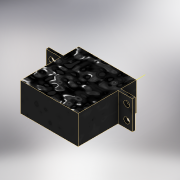
# Autodesk Inventor part: Servo
Saved by Autodesk Inventor 2021 (Build 250183000, 183)
## iProperties
Created: 2024-03-17
Part Number: Servo
Material: PLA
Document SubType Name: Modeling
Designer: Martin
Density: 1.27 g/cm^3
Appearance: PLA
Mass: 42.079 g
Surface Area: 72.9716 cm^2
Volume: 33.1331 cm^3
Author: Martin
Autodesk Inventor part; units mm, degrees
ref_plane "YZ Plane" through (0, 0, 0) normal (1, 0, 0) x (0, 1, 0)
ref_plane "XZ Plane" through (0, 0, 0) normal (0, 1, 0) x (-1, 0, 0)
ref_plane "XY Plane" through (0, 0, 0) normal (0, 0, 1) x (1, 0, 0)
sketch "Sketch1" plane through (0, 0, 0) normal (0, 1, 0) x (-1, 0, 0)
  line L0 (-20, 0) -> (20, 0)
  line L1 (20, 0) -> (20, -40.5)
  line L2 (20, -40.5) -> (-20, -40.5)
  line L3 (-20, -40.5) -> (-20, 0)
  point P0 (0, 0)
  point P1 (0, -40.5)
  dimension "d0" = 40
  dimension "d1" = 40.5
  constraints: 8 end point, 2 parallel, 1 horizontal, 1 midpoint, 1 perpendicular
  measures "d0" distance of L1.end L2.end
  measures "d1" distance of L0.end L1.end
extrude "Extrusion1" add sketch "Sketch1" along normal blind 20
sketch "Sketch2" plane through (20, 0, 0) normal (1, 0, 0) x (0, 0, -1)
  line L0 (27.7, 20) -> (29.7, 20)
  line L1 (29.7, 20) -> (29.7, 0)
  line L2 (29.7, 0) -> (27.7, 0)
  line L3 (27.7, 0) -> (27.7, 20)
  line L4 (40.5, 0) -> (40.5, 20) projected
  line L5 (0, 0) -> (0, 20) projected
  dimension "d4" = 2
  dimension "d31" = 27.7
  constraints: 8 end point, 2 parallel, 1 horizontal, 1 perpendicular
  measures "d4" distance of L1.end L2.end
  measures "d31" distance between parallel lines of L3 L5
extrude "Extrusion2" add sketch "Sketch2" along normal blind 10
sketch "Sketch3" plane through (20, 0, -29.7) normal (0, 0, -1) x (-1, 0, 0)
  circle A0 centre (-6, 15) radius 2
  line L0 (-10, 20) -> (-10, 0) projected
  line L1 (-10, 10) -> (0, 10)
  circle A1 centre (-6, 5) radius 2
  point P0 (20, 0)
  point P1 (-10, 5)
  point P2 (-8, 3.2679)
  dimension "d9" = 4
  dimension "d13" = 5
  dimension "d32" = 4
  constraints: 2 centre point, 2 end point, 1 horizontal, 1 midpoint, 1 symmetric about line, 1 other
  measures "d9" diameter of A0
  measures "d13" distance from line of A0.centre L1
  measures "d32" distance from line of L0 A0.centre
extrude "Extrusion3" cut sketch "Sketch3" against normal up to next
sketch "Sketch4" plane through (20, 0, -40.5) normal (0, 0, -1) x (-1, 0, 0)
  circle A0 centre (10, 10) radius 3
  line L0 (0, 0) -> (0, 20) projected
  line L1 (0, 20) -> (40, 20) projected
  point P0 (20, 0)
  dimension "d16" = 6
  dimension "d17" = 10
  dimension "d18" = 10
  constraints: 1 centre point
  measures "d16" diameter of A0
  measures "d17" distance from line of L0 A0.centre
  measures "d18" distance from line of L1 A0.centre
extrude "Extrusion4" add sketch "Sketch4" along normal blind 6
sketch "Sketch5" plane through (10, 10, -46.5) normal (0, 0, -1) x (-1, 0, 0)
  circle A0 centre (0, 0) radius 3 projected
  line L0 (2.75, -0.1872) -> (3.25, -0.1872)
  line L1 (3.25, -0.1872) -> (3.25, 0.1872)
  line L2 (3.25, 0.1872) -> (2.75, 0.1872)
  line L3 (2.75, 0.1872) -> (2.75, -0.1872)
  line L4 (2.75, -0.1872) -> (3.25, 0.1872) construction
  line L5 (3.25, -0.1872) -> (2.75, 0.1872) construction
  line L6 (2.5575, 1.0279) -> (2.6733, 0.6717)
  line L7 (3.0331, 1.1824) -> (2.5575, 1.0279)
  line L8 (3.1488, 0.8262) -> (3.0331, 1.1824)
  line L9 (2.6733, 0.6717) -> (3.1488, 0.8262)
  line L10 (2.1147, 1.7679) -> (2.3348, 1.4649)
  line L11 (2.5193, 2.0618) -> (2.1147, 1.7679)
  line L12 (2.7394, 1.7588) -> (2.5193, 2.0618)
  line L13 (2.3348, 1.4649) -> (2.7394, 1.7588)
  line L14 (1.4649, 2.3348) -> (1.7679, 2.1147)
  line L15 (1.7588, 2.7394) -> (1.4649, 2.3348)
  line L16 (2.0618, 2.5193) -> (1.7588, 2.7394)
  line L17 (1.7679, 2.1147) -> (2.0618, 2.5193)
  line L18 (0.6717, 2.6733) -> (1.0279, 2.5575)
  line L19 (0.8262, 3.1488) -> (0.6717, 2.6733)
  line L20 (1.1824, 3.0331) -> (0.8262, 3.1488)
  line L21 (1.0279, 2.5575) -> (1.1824, 3.0331)
  line L22 (-0.1872, 2.75) -> (0.1872, 2.75)
  line L23 (-0.1872, 3.25) -> (-0.1872, 2.75)
  line L24 (0.1872, 3.25) -> (-0.1872, 3.25)
  line L25 (0.1872, 2.75) -> (0.1872, 3.25)
  line L26 (-1.0279, 2.5575) -> (-0.6717, 2.6733)
  line L27 (-1.1824, 3.0331) -> (-1.0279, 2.5575)
  line L28 (-0.8262, 3.1488) -> (-1.1824, 3.0331)
  line L29 (-0.6717, 2.6733) -> (-0.8262, 3.1488)
  line L30 (-1.7679, 2.1147) -> (-1.4649, 2.3348)
  line L31 (-2.0618, 2.5193) -> (-1.7679, 2.1147)
  line L32 (-1.7588, 2.7394) -> (-2.0618, 2.5193)
  line L33 (-1.4649, 2.3348) -> (-1.7588, 2.7394)
  line L34 (-2.3348, 1.4649) -> (-2.1147, 1.7679)
  line L35 (-2.7394, 1.7588) -> (-2.3348, 1.4649)
  line L36 (-2.5193, 2.0618) -> (-2.7394, 1.7588)
  line L37 (-2.1147, 1.7679) -> (-2.5193, 2.0618)
  line L38 (-2.6733, 0.6717) -> (-2.5575, 1.0279)
  line L39 (-3.1488, 0.8262) -> (-2.6733, 0.6717)
  line L40 (-3.0331, 1.1824) -> (-3.1488, 0.8262)
  line L41 (-2.5575, 1.0279) -> (-3.0331, 1.1824)
  line L42 (-2.75, -0.1872) -> (-2.75, 0.1872)
  line L43 (-3.25, -0.1872) -> (-2.75, -0.1872)
  line L44 (-3.25, 0.1872) -> (-3.25, -0.1872)
  line L45 (-2.75, 0.1872) -> (-3.25, 0.1872)
  line L46 (-2.5575, -1.0279) -> (-2.6733, -0.6717)
  line L47 (-3.0331, -1.1824) -> (-2.5575, -1.0279)
  line L48 (-3.1488, -0.8262) -> (-3.0331, -1.1824)
  line L49 (-2.6733, -0.6717) -> (-3.1488, -0.8262)
  line L50 (-2.1147, -1.7679) -> (-2.3348, -1.4649)
  line L51 (-2.5193, -2.0618) -> (-2.1147, -1.7679)
  line L52 (-2.7394, -1.7588) -> (-2.5193, -2.0618)
  line L53 (-2.3348, -1.4649) -> (-2.7394, -1.7588)
  line L54 (-1.4649, -2.3348) -> (-1.7679, -2.1147)
  line L55 (-1.7588, -2.7394) -> (-1.4649, -2.3348)
  line L56 (-2.0618, -2.5193) -> (-1.7588, -2.7394)
  line L57 (-1.7679, -2.1147) -> (-2.0618, -2.5193)
  line L58 (-0.6717, -2.6733) -> (-1.0279, -2.5575)
  line L59 (-0.8262, -3.1488) -> (-0.6717, -2.6733)
  line L60 (-1.1824, -3.0331) -> (-0.8262, -3.1488)
  line L61 (-1.0279, -2.5575) -> (-1.1824, -3.0331)
  line L62 (0.1872, -2.75) -> (-0.1872, -2.75)
  line L63 (0.1872, -3.25) -> (0.1872, -2.75)
  line L64 (-0.1872, -3.25) -> (0.1872, -3.25)
  line L65 (-0.1872, -2.75) -> (-0.1872, -3.25)
  line L66 (1.0279, -2.5575) -> (0.6717, -2.6733)
  line L67 (1.1824, -3.0331) -> (1.0279, -2.5575)
  line L68 (0.8262, -3.1488) -> (1.1824, -3.0331)
  line L69 (0.6717, -2.6733) -> (0.8262, -3.1488)
  line L70 (1.7679, -2.1147) -> (1.4649, -2.3348)
  line L71 (2.0618, -2.5193) -> (1.7679, -2.1147)
  line L72 (1.7588, -2.7394) -> (2.0618, -2.5193)
  line L73 (1.4649, -2.3348) -> (1.7588, -2.7394)
  line L74 (2.3348, -1.4649) -> (2.1147, -1.7679)
  line L75 (2.7394, -1.7588) -> (2.3348, -1.4649)
  line L76 (2.5193, -2.0618) -> (2.7394, -1.7588)
  line L77 (2.1147, -1.7679) -> (2.5193, -2.0618)
  line L78 (2.6733, -0.6717) -> (2.5575, -1.0279)
  line L79 (3.1488, -0.8262) -> (2.6733, -0.6717)
  line L80 (3.0331, -1.1824) -> (3.1488, -0.8262)
  line L81 (2.5575, -1.0279) -> (3.0331, -1.1824)
  point P0 (10, -10)
  point P1 (3, 0)
  dimension "d21" = 0.5
  dimension "d24" = 360
  constraints: 164 end point, 2 midpoint, 2 parallel, 1 horizontal, 1 horizontal alignment, 1 perpendicular, 162 other
  measures "d21" distance of L2.end L1.end
extrude "Extrusion5" cut sketch "Sketch5" against normal up to surface (6 mm away) contours A0 L0 L3 L2 | A0 L2 L1 L0
pattern_circular "Circular Pattern1" count 20 over 360 about axis through (10, 10, -46.5) along (0, 0, -1) of "Extrusion5"
mirror "Mirror1" about plane through (0, 0, 0) normal (1, 0, 0) of "Extrusion2", "Extrusion3"
body "Solid1"
